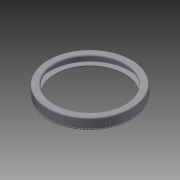
# Autodesk Inventor part: tire
Saved by Autodesk Inventor 2014 (Build 180170000, 170)
## iProperties
Created: 2013-06-25
Part Number: tire
Material: Generisch
Document SubType Name: Modeling
Designer: Felix
Density: 1 g/cm^3
Appearance: Vorgabe
Author: Felix
Autodesk Inventor part; units mm, degrees
ref_plane "YZ Plane" through (0, 0, 0) normal (1, 0, 0) x (0, 1, 0)
ref_plane "XZ Plane" through (0, 0, 0) normal (0, 1, 0) x (-1, 0, 0)
sketch "Skizze1" plane through (0, 0, 0) normal (0, 0, 1) x (1, 0, 0)
  circle A0 centre (0, 0) radius 30
  circle A1 centre (0, 0) radius 25
  dimension "d0" = 60
  dimension "d1" = 50
  constraints: 2 centre point, 2 coincident
  measures "d0" diameter of A0
  measures "d1" diameter of A1
extrude "Extrusion1" add sketch "Skizze1" along normal blind 8
ref_plane "Arbeitsebene3" through (0, 0, 4) normal (0, 0, -1) x (-1, 0, 0)
shell "Hülle1" thickness 1.5 removed faces 1 at (24.9189, -2.0117, 5.3333)
sketch "Skizze4" plane through (0, 0, 4) normal (0, 0, -1) x (-1, 0, 0)
  circle A0 centre (0, 0) radius 30
  line L0 (-17.9589, 24.0308) -> (-18.7498, 23.4189)
  line L1 (-18.7498, 23.4189) -> (-18.4438, 23.0234)
  line L2 (-18.4438, 23.0234) -> (-17.6529, 23.6353)
  line L3 (-17.6529, 23.6353) -> (-17.9589, 24.0308)
  dimension "d11" = 1
  dimension "d14" = 0.5
  constraints: 8 end point, 2 parallel, 2 point on circle, 1 centre point, 1 perpendicular
  measures "d11" distance of L0.start L0.end
  measures "d14" distance of L0.end L1.end
extrude "Extrusion3" cut sketch "Skizze4" along normal mid plane 6 contours L0 A0 | L3 L2 L1 L0
pattern_circular "Runde Anordnung1" count 110 over 360 about axis through (0, 0, -10) along (0, 0, 1) of "Extrusion3"
fillet "Rundung1" radius 1 2 edges at (-30, 0, 8) (-30, 0, 0)
fillet "Rundung2" radius 1 2 edges at (-25, 0, 8) (-25, 0, 0)
